Autodesk Fusion 360 part; units mm, degrees
(part 2 of 2)
  spline S384 degree 2 poles (40.9942, 8.1842) (40.8646, 8.1842) (40.7546, 8.116) knots 0 0 0 1 1 1
  spline S385 degree 2 poles (40.7546, 8.116) (40.6446, 8.0477) (40.5952, 7.9164) knots 0 0 0 1 1 1
  spline S386 degree 2 poles (40.5952, 7.9164) (40.5457, 7.7851) (40.5457, 7.5379) knots 0 0 0 1 1 1
  line L215 (40.5457, 7.5379) -> (40.5457, 6.5982)
  line L216 (40.5457, 6.5982) -> (40.2387, 6.5982)
  line L217 (44.3878, 7.1814) -> (44.705, 7.1422)
  spline S387 degree 2 poles (44.705, 7.1422) (44.6299, 6.8643) (44.427, 6.7108) knots 0 0 0 1 1 1
  spline S388 degree 2 poles (44.427, 6.7108) (44.2241, 6.5573) (43.9086, 6.5573) knots 0 0 0 1 1 1
  spline S389 degree 2 poles (43.9086, 6.5573) (43.5113, 6.5573) (43.2785, 6.802) knots 0 0 0 1 1 1
  spline S390 degree 2 poles (43.2785, 6.802) (43.0457, 7.0467) (43.0457, 7.4884) knots 0 0 0 1 1 1
  spline S391 degree 2 poles (43.0457, 7.4884) (43.0457, 7.9454) (43.281, 8.1978) knots 0 0 0 1 1 1
  spline S392 degree 2 poles (43.281, 8.1978) (43.5164, 8.4502) (43.8915, 8.4502) knots 0 0 0 1 1 1
  spline S393 degree 2 poles (43.8915, 8.4502) (44.2548, 8.4502) (44.485, 8.2029) knots 0 0 0 1 1 1
  spline S394 degree 2 poles (44.485, 8.2029) (44.7152, 7.9557) (44.7152, 7.5072) knots 0 0 0 1 1 1
  spline S395 degree 2 poles (44.7152, 7.5072) (44.7152, 7.4799) (44.7135, 7.4253) knots 0 0 0 1 1 1
  line L218 (44.7135, 7.4253) -> (43.3629, 7.4253)
  spline S396 degree 2 poles (43.3629, 7.4253) (43.3799, 7.1269) (43.5317, 6.9683) knots 0 0 0 1 1 1
  spline S397 degree 2 poles (43.5317, 6.9683) (43.6835, 6.8097) (43.9103, 6.8097) knots 0 0 0 1 1 1
  spline S398 degree 2 poles (43.9103, 6.8097) (44.0791, 6.8097) (44.1985, 6.8984) knots 0 0 0 1 1 1
  spline S399 degree 2 poles (44.1985, 6.8984) (44.3179, 6.987) (44.3878, 7.1814) knots 0 0 0 1 1 1
  line L219 (43.3799, 7.6777) -> (44.3912, 7.6777)
  spline S400 degree 2 poles (44.3912, 7.6777) (44.3707, 7.9062) (44.2752, 8.0205) knots 0 0 0 1 1 1
  spline S401 degree 2 poles (44.2752, 8.0205) (44.1286, 8.1978) (43.895, 8.1978) knots 0 0 0 1 1 1
  spline S402 degree 2 poles (43.895, 8.1978) (43.6835, 8.1978) (43.5394, 8.0563) knots 0 0 0 1 1 1
  spline S403 degree 2 poles (43.5394, 8.0563) (43.3953, 7.9147) (43.3799, 7.6777) knots 0 0 0 1 1 1
  line L220 (45.0904, 6.5982) -> (45.0904, 8.4093)
  line L221 (45.0904, 8.4093) -> (45.3666, 8.4093)
  line L222 (45.3666, 8.4093) -> (45.3666, 8.1518)
  spline S404 degree 2 poles (45.3666, 8.1518) (45.5662, 8.4502) (45.943, 8.4502) knots 0 0 0 1 1 1
  spline S405 degree 2 poles (45.943, 8.4502) (46.1068, 8.4502) (46.244, 8.3914) knots 0 0 0 1 1 1
  spline S406 degree 2 poles (46.244, 8.3914) (46.3813, 8.3325) (46.4495, 8.237) knots 0 0 0 1 1 1
  spline S407 degree 2 poles (46.4495, 8.237) (46.5177, 8.1415) (46.545, 8.0102) knots 0 0 0 1 1 1
  spline S408 degree 2 poles (46.545, 8.0102) (46.5621, 7.925) (46.5621, 7.7118) knots 0 0 0 1 1 1
  line L223 (46.5621, 7.7118) -> (46.5621, 6.5982)
  line L224 (46.5621, 6.5982) -> (46.2551, 6.5982)
  line L225 (46.2551, 6.5982) -> (46.2551, 7.6999)
  spline S409 degree 2 poles (46.2551, 7.6999) (46.2551, 7.8874) (46.2193, 7.9804) knots 0 0 0 1 1 1
  spline S410 degree 2 poles (46.2193, 7.9804) (46.1835, 8.0733) (46.0923, 8.1288) knots 0 0 0 1 1 1
  spline S411 degree 2 poles (46.0923, 8.1288) (46.001, 8.1842) (45.8782, 8.1842) knots 0 0 0 1 1 1
  spline S412 degree 2 poles (45.8782, 8.1842) (45.6821, 8.1842) (45.5397, 8.0597) knots 0 0 0 1 1 1
  spline S413 degree 2 poles (45.5397, 8.0597) (45.3973, 7.9352) (45.3973, 7.5873) knots 0 0 0 1 1 1
  line L226 (45.3973, 7.5873) -> (45.3973, 6.5982)
  line L227 (45.3973, 6.5982) -> (45.0904, 6.5982)
  line L228 (47.7029, 6.8728) -> (47.7473, 6.6016)
  spline S414 degree 2 poles (47.7473, 6.6016) (47.6177, 6.5744) (47.5153, 6.5744) knots 0 0 0 1 1 1
  spline S415 degree 2 poles (47.5153, 6.5744) (47.3482, 6.5744) (47.2561, 6.6272) knots 0 0 0 1 1 1
  spline S416 degree 2 poles (47.2561, 6.6272) (47.1641, 6.6801) (47.1265, 6.7662) knots 0 0 0 1 1 1
  spline S417 degree 2 poles (47.1265, 6.7662) (47.089, 6.8523) (47.089, 7.1286) knots 0 0 0 1 1 1
  line L229 (47.089, 7.1286) -> (47.089, 8.1705)
  line L230 (47.089, 8.1705) -> (46.8639, 8.1705)
  line L231 (46.8639, 8.1705) -> (46.8639, 8.4093)
  line L232 (46.8639, 8.4093) -> (47.089, 8.4093)
  line L233 (47.089, 8.4093) -> (47.089, 8.8578)
  line L234 (47.089, 8.8578) -> (47.3943, 9.042)
  line L235 (47.3943, 9.042) -> (47.3943, 8.4093)
  line L236 (47.3943, 8.4093) -> (47.7029, 8.4093)
  line L237 (47.7029, 8.4093) -> (47.7029, 8.1705)
  line L238 (47.7029, 8.1705) -> (47.3943, 8.1705)
  line L239 (47.3943, 8.1705) -> (47.3943, 7.1115)
  spline S418 degree 2 poles (47.3943, 7.1115) (47.3943, 6.9802) (47.4105, 6.9427) knots 0 0 0 1 1 1
  spline S419 degree 2 poles (47.4105, 6.9427) (47.4267, 6.9052) (47.4633, 6.883) knots 0 0 0 1 1 1
  spline S420 degree 2 poles (47.4633, 6.883) (47.5, 6.8608) (47.5682, 6.8608) knots 0 0 0 1 1 1
  spline S421 degree 2 poles (47.5682, 6.8608) (47.6194, 6.8608) (47.7029, 6.8728) knots 0 0 0 1 1 1
  line L240 (11.8426, 2.6965) -> (11.2884, 4.5075)
  line L241 (11.2884, 4.5075) -> (11.6056, 4.5075)
  line L242 (11.6056, 4.5075) -> (11.8938, 3.4621)
  line L243 (11.8938, 3.4621) -> (12.0012, 3.0733)
  spline S422 degree 2 poles (12.0012, 3.0733) (12.008, 3.1023) (12.095, 3.4468) knots 0 0 0 1 1 1
  line L244 (12.095, 3.4468) -> (12.3832, 4.5075)
  line L245 (12.3832, 4.5075) -> (12.6987, 4.5075)
  line L246 (12.6987, 4.5075) -> (12.9698, 3.457)
  line L247 (12.9698, 3.457) -> (13.0602, 3.1108)
  line L248 (13.0602, 3.1108) -> (13.1642, 3.4604)
  line L249 (13.1642, 3.4604) -> (13.4746, 4.5075)
  line L250 (13.4746, 4.5075) -> (13.773, 4.5075)
  line L251 (13.773, 4.5075) -> (13.2069, 2.6965)
  line L252 (13.2069, 2.6965) -> (12.888, 2.6965)
  line L253 (12.888, 2.6965) -> (12.5998, 3.781)
  line L254 (12.5998, 3.781) -> (12.5298, 4.0897)
  line L255 (12.5298, 4.0897) -> (12.1632, 2.6965)
  line L256 (12.1632, 2.6965) -> (11.8426, 2.6965)
  line L257 (14.3648, 2.6965) -> (13.8105, 4.5075)
  line L258 (13.8105, 4.5075) -> (14.1277, 4.5075)
  line L259 (14.1277, 4.5075) -> (14.4159, 3.4621)
  line L260 (14.4159, 3.4621) -> (14.5234, 3.0733)
  spline S423 degree 2 poles (14.5234, 3.0733) (14.5302, 3.1023) (14.6172, 3.4468) knots 0 0 0 1 1 1
  line L261 (14.6172, 3.4468) -> (14.9054, 4.5075)
  line L262 (14.9054, 4.5075) -> (15.2208, 4.5075)
  line L263 (15.2208, 4.5075) -> (15.492, 3.457)
  line L264 (15.492, 3.457) -> (15.5824, 3.1108)
  line L265 (15.5824, 3.1108) -> (15.6864, 3.4604)
  line L266 (15.6864, 3.4604) -> (15.9968, 4.5075)
  line L267 (15.9968, 4.5075) -> (16.2952, 4.5075)
  line L268 (16.2952, 4.5075) -> (15.729, 2.6965)
  line L269 (15.729, 2.6965) -> (15.4101, 2.6965)
  line L270 (15.4101, 2.6965) -> (15.1219, 3.781)
  line L271 (15.1219, 3.781) -> (15.052, 4.0897)
  line L272 (15.052, 4.0897) -> (14.6854, 2.6965)
  line L273 (14.6854, 2.6965) -> (14.3648, 2.6965)
  line L274 (16.8869, 2.6965) -> (16.3327, 4.5075)
  line L275 (16.3327, 4.5075) -> (16.6499, 4.5075)
  line L276 (16.6499, 4.5075) -> (16.9381, 3.4621)
  line L277 (16.9381, 3.4621) -> (17.0455, 3.0733)
  spline S424 degree 2 poles (17.0455, 3.0733) (17.0524, 3.1023) (17.1393, 3.4468) knots 0 0 0 1 1 1
  line L278 (17.1393, 3.4468) -> (17.4275, 4.5075)
  line L279 (17.4275, 4.5075) -> (17.743, 4.5075)
  line L280 (17.743, 4.5075) -> (18.0142, 3.457)
  line L281 (18.0142, 3.457) -> (18.1045, 3.1108)
  line L282 (18.1045, 3.1108) -> (18.2086, 3.4604)
  line L283 (18.2086, 3.4604) -> (18.5189, 4.5075)
  line L284 (18.5189, 4.5075) -> (18.8174, 4.5075)
  line L285 (18.8174, 4.5075) -> (18.2512, 2.6965)
  line L286 (18.2512, 2.6965) -> (17.9323, 2.6965)
  line L287 (17.9323, 2.6965) -> (17.6441, 3.781)
  line L288 (17.6441, 3.781) -> (17.5742, 4.0897)
  line L289 (17.5742, 4.0897) -> (17.2075, 2.6965)
  line L290 (17.2075, 2.6965) -> (16.8869, 2.6965)
  line L291 (18.9691, 2.6965) -> (18.9691, 3.046)
  line L292 (18.9691, 3.046) -> (19.3187, 3.046)
  line L293 (19.3187, 3.046) -> (19.3187, 2.6965)
  line L294 (19.3187, 2.6965) -> (18.9691, 2.6965)
  line L295 (19.8525, 2.6965) -> (19.8525, 4.5075)
  line L296 (19.8525, 4.5075) -> (20.127, 4.5075)
  line L297 (20.127, 4.5075) -> (20.127, 4.2534)
  spline S425 degree 2 poles (20.127, 4.2534) (20.2123, 4.3864) (20.3539, 4.4674) knots 0 0 0 1 1 1
  spline S426 degree 2 poles (20.3539, 4.4674) (20.4954, 4.5484) (20.6762, 4.5484) knots 0 0 0 1 1 1
  spline S427 degree 2 poles (20.6762, 4.5484) (20.8774, 4.5484) (21.0061, 4.4649) knots 0 0 0 1 1 1
  spline S428 degree 2 poles (21.0061, 4.4649) (21.1349, 4.3813) (21.1878, 4.2312) knots 0 0 0 1 1 1
  spline S429 degree 2 poles (21.1878, 4.2312) (21.4026, 4.5484) (21.7471, 4.5484) knots 0 0 0 1 1 1
  spline S430 degree 2 poles (21.7471, 4.5484) (22.0165, 4.5484) (22.1615, 4.3992) knots 0 0 0 1 1 1
  spline S431 degree 2 poles (22.1615, 4.3992) (22.3064, 4.25) (22.3064, 3.9396) knots 0 0 0 1 1 1
  line L298 (22.3064, 3.9396) -> (22.3064, 2.6965)
  line L299 (22.3064, 2.6965) -> (22.0012, 2.6965)
  line L300 (22.0012, 2.6965) -> (22.0012, 3.8373)
  spline S432 degree 2 poles (22.0012, 3.8373) (22.0012, 4.0215) (21.9713, 4.1025) knots 0 0 0 1 1 1
  spline S433 degree 2 poles (21.9713, 4.1025) (21.9415, 4.1835) (21.8631, 4.2329) knots 0 0 0 1 1 1
  spline S434 degree 2 poles (21.8631, 4.2329) (21.7846, 4.2824) (21.6789, 4.2824) knots 0 0 0 1 1 1
  spline S435 degree 2 poles (21.6789, 4.2824) (21.4879, 4.2824) (21.3617, 4.1554) knots 0 0 0 1 1 1
  spline S436 degree 2 poles (21.3617, 4.1554) (21.2355, 4.0283) (21.2355, 3.7486) knots 0 0 0 1 1 1
  line L301 (21.2355, 3.7486) -> (21.2355, 2.6965)
  line L302 (21.2355, 2.6965) -> (20.9285, 2.6965)
  line L303 (20.9285, 2.6965) -> (20.9285, 3.8731)
  spline S437 degree 2 poles (20.9285, 3.8731) (20.9285, 4.0778) (20.8535, 4.1801) knots 0 0 0 1 1 1
  spline S438 degree 2 poles (20.8535, 4.1801) (20.7785, 4.2824) (20.6079, 4.2824) knots 0 0 0 1 1 1
  spline S439 degree 2 poles (20.6079, 4.2824) (20.4783, 4.2824) (20.3683, 4.2142) knots 0 0 0 1 1 1
  spline S440 degree 2 poles (20.3683, 4.2142) (20.2584, 4.146) (20.2089, 4.0147) knots 0 0 0 1 1 1
  spline S441 degree 2 poles (20.2089, 4.0147) (20.1594, 3.8834) (20.1594, 3.6361) knots 0 0 0 1 1 1
  line L304 (20.1594, 3.6361) -> (20.1594, 2.6965)
  line L305 (20.1594, 2.6965) -> (19.8525, 2.6965)
  spline S442 degree 2 poles (22.6475, 3.602) (22.6475, 4.105) (22.9272, 4.3472) knots 0 0 0 1 1 1
  spline S443 degree 2 poles (22.9272, 4.3472) (23.1608, 4.5484) (23.4968, 4.5484) knots 0 0 0 1 1 1
  spline S444 degree 2 poles (23.4968, 4.5484) (23.8702, 4.5484) (24.1073, 4.3037) knots 0 0 0 1 1 1
  spline S445 degree 2 poles (24.1073, 4.3037) (24.3443, 4.059) (24.3443, 3.6276) knots 0 0 0 1 1 1
  spline S446 degree 2 poles (24.3443, 3.6276) (24.3443, 3.278) (24.2394, 3.0776) knots 0 0 0 1 1 1
  spline S447 degree 2 poles (24.2394, 3.0776) (24.1345, 2.8772) (23.9342, 2.7664) knots 0 0 0 1 1 1
  spline S448 degree 2 poles (23.9342, 2.7664) (23.7338, 2.6555) (23.4968, 2.6555) knots 0 0 0 1 1 1
  spline S449 degree 2 poles (23.4968, 2.6555) (23.1165, 2.6555) (22.882, 2.8994) knots 0 0 0 1 1 1
  spline S450 degree 2 poles (22.882, 2.8994) (22.6475, 3.1432) (22.6475, 3.602) knots 0 0 0 1 1 1
  spline S451 degree 2 poles (22.963, 3.602) (22.963, 3.2541) (23.1148, 3.081) knots 0 0 0 1 1 1
  spline S452 degree 2 poles (23.1148, 3.081) (23.2665, 2.9079) (23.4968, 2.9079) knots 0 0 0 1 1 1
  spline S453 degree 2 poles (23.4968, 2.9079) (23.7253, 2.9079) (23.877, 3.0819) knots 0 0 0 1 1 1
  spline S454 degree 2 poles (23.877, 3.0819) (24.0288, 3.2558) (24.0288, 3.6122) knots 0 0 0 1 1 1
  spline S455 degree 2 poles (24.0288, 3.6122) (24.0288, 3.9482) (23.8762, 4.1212) knots 0 0 0 1 1 1
  spline S456 degree 2 poles (23.8762, 4.1212) (23.7236, 4.2943) (23.4968, 4.2943) knots 0 0 0 1 1 1
  spline S457 degree 2 poles (23.4968, 4.2943) (23.2665, 4.2943) (23.1148, 4.1221) knots 0 0 0 1 1 1
  spline S458 degree 2 poles (23.1148, 4.1221) (22.963, 3.9499) (22.963, 3.602) knots 0 0 0 1 1 1
  line L306 (24.7041, 2.6965) -> (24.7041, 4.5075)
  line L307 (24.7041, 4.5075) -> (24.9804, 4.5075)
  line L308 (24.9804, 4.5075) -> (24.9804, 4.25)
  spline S459 degree 2 poles (24.9804, 4.25) (25.1799, 4.5484) (25.5568, 4.5484) knots 0 0 0 1 1 1
  spline S460 degree 2 poles (25.5568, 4.5484) (25.7205, 4.5484) (25.8578, 4.4896) knots 0 0 0 1 1 1
  spline S461 degree 2 poles (25.8578, 4.4896) (25.9951, 4.4308) (26.0633, 4.3353) knots 0 0 0 1 1 1
  spline S462 degree 2 poles (26.0633, 4.3353) (26.1315, 4.2398) (26.1588, 4.1085) knots 0 0 0 1 1 1
  spline S463 degree 2 poles (26.1588, 4.1085) (26.1758, 4.0232) (26.1758, 3.81) knots 0 0 0 1 1 1
  line L309 (26.1758, 3.81) -> (26.1758, 2.6965)
  line L310 (26.1758, 2.6965) -> (25.8689, 2.6965)
  line L311 (25.8689, 2.6965) -> (25.8689, 3.7981)
  spline S464 degree 2 poles (25.8689, 3.7981) (25.8689, 3.9857) (25.833, 4.0786) knots 0 0 0 1 1 1
  spline S465 degree 2 poles (25.833, 4.0786) (25.7972, 4.1716) (25.706, 4.227) knots 0 0 0 1 1 1
  spline S466 degree 2 poles (25.706, 4.227) (25.6148, 4.2824) (25.492, 4.2824) knots 0 0 0 1 1 1
  spline S467 degree 2 poles (25.492, 4.2824) (25.2959, 4.2824) (25.1535, 4.1579) knots 0 0 0 1 1 1
  spline S468 degree 2 poles (25.1535, 4.1579) (25.0111, 4.0334) (25.0111, 3.6855) knots 0 0 0 1 1 1
  line L312 (25.0111, 3.6855) -> (25.0111, 2.6965)
  line L313 (25.0111, 2.6965) -> (24.7041, 2.6965)
  line L314 (27.3167, 2.971) -> (27.361, 2.6999)
  spline S469 degree 2 poles (27.361, 2.6999) (27.2314, 2.6726) (27.1291, 2.6726) knots 0 0 0 1 1 1
  spline S470 degree 2 poles (27.1291, 2.6726) (26.962, 2.6726) (26.8699, 2.7254) knots 0 0 0 1 1 1
  spline S471 degree 2 poles (26.8699, 2.7254) (26.7778, 2.7783) (26.7403, 2.8644) knots 0 0 0 1 1 1
  spline S472 degree 2 poles (26.7403, 2.8644) (26.7028, 2.9505) (26.7028, 3.2268) knots 0 0 0 1 1 1
  line L315 (26.7028, 3.2268) -> (26.7028, 4.2688)
  line L316 (26.7028, 4.2688) -> (26.4777, 4.2688)
  line L317 (26.4777, 4.2688) -> (26.4777, 4.5075)
  line L318 (26.4777, 4.5075) -> (26.7028, 4.5075)
  line L319 (26.7028, 4.5075) -> (26.7028, 4.956)
  line L320 (26.7028, 4.956) -> (27.008, 5.1402)
  line L321 (27.008, 5.1402) -> (27.008, 4.5075)
  line L322 (27.008, 4.5075) -> (27.3167, 4.5075)
  line L323 (27.3167, 4.5075) -> (27.3167, 4.2688)
  line L324 (27.3167, 4.2688) -> (27.008, 4.2688)
  line L325 (27.008, 4.2688) -> (27.008, 3.2098)
  spline S473 degree 2 poles (27.008, 3.2098) (27.008, 3.0784) (27.0242, 3.0409) knots 0 0 0 1 1 1
  spline S474 degree 2 poles (27.0242, 3.0409) (27.0404, 3.0034) (27.0771, 2.9812) knots 0 0 0 1 1 1
  spline S475 degree 2 poles (27.0771, 2.9812) (27.1137, 2.9591) (27.182, 2.9591) knots 0 0 0 1 1 1
  spline S476 degree 2 poles (27.182, 2.9591) (27.2331, 2.9591) (27.3167, 2.971) knots 0 0 0 1 1 1
  line L326 (28.8566, 3.2797) -> (29.1738, 3.2405)
  spline S477 degree 2 poles (29.1738, 3.2405) (29.0987, 2.9625) (28.8958, 2.809) knots 0 0 0 1 1 1
  spline S478 degree 2 poles (28.8958, 2.809) (28.6929, 2.6555) (28.3774, 2.6555) knots 0 0 0 1 1 1
  spline S479 degree 2 poles (28.3774, 2.6555) (27.98, 2.6555) (27.7473, 2.9002) knots 0 0 0 1 1 1
  spline S480 degree 2 poles (27.7473, 2.9002) (27.5145, 3.145) (27.5145, 3.5866) knots 0 0 0 1 1 1
  spline S481 degree 2 poles (27.5145, 3.5866) (27.5145, 4.0437) (27.7498, 4.296) knots 0 0 0 1 1 1
  spline S482 degree 2 poles (27.7498, 4.296) (27.9852, 4.5484) (28.3603, 4.5484) knots 0 0 0 1 1 1
  spline S483 degree 2 poles (28.3603, 4.5484) (28.7236, 4.5484) (28.9538, 4.3012) knots 0 0 0 1 1 1
  spline S484 degree 2 poles (28.9538, 4.3012) (29.184, 4.0539) (29.184, 3.6054) knots 0 0 0 1 1 1
  spline S485 degree 2 poles (29.184, 3.6054) (29.184, 3.5781) (29.1823, 3.5235) knots 0 0 0 1 1 1
  line L327 (29.1823, 3.5235) -> (27.8317, 3.5235)
  spline S486 degree 2 poles (27.8317, 3.5235) (27.8487, 3.2251) (28.0005, 3.0665) knots 0 0 0 1 1 1
  spline S487 degree 2 poles (28.0005, 3.0665) (28.1523, 2.9079) (28.3791, 2.9079) knots 0 0 0 1 1 1
  spline S488 degree 2 poles (28.3791, 2.9079) (28.5479, 2.9079) (28.6673, 2.9966) knots 0 0 0 1 1 1
  spline S489 degree 2 poles (28.6673, 2.9966) (28.7867, 3.0853) (28.8566, 3.2797) knots 0 0 0 1 1 1
  line L328 (27.8487, 3.7759) -> (28.86, 3.7759)
  spline S490 degree 2 poles (28.86, 3.7759) (28.8395, 4.0044) (28.744, 4.1187) knots 0 0 0 1 1 1
  spline S491 degree 2 poles (28.744, 4.1187) (28.5974, 4.296) (28.3637, 4.296) knots 0 0 0 1 1 1
  spline S492 degree 2 poles (28.3637, 4.296) (28.1523, 4.296) (28.0082, 4.1545) knots 0 0 0 1 1 1
  spline S493 degree 2 poles (28.0082, 4.1545) (27.8641, 4.013) (27.8487, 3.7759) knots 0 0 0 1 1 1
  line L329 (30.7341, 2.6965) -> (30.7341, 2.925)
  spline S494 degree 2 poles (30.7341, 2.925) (30.5619, 2.6555) (30.2277, 2.6555) knots 0 0 0 1 1 1
  spline S495 degree 2 poles (30.2277, 2.6555) (30.0111, 2.6555) (29.8295, 2.7749) knots 0 0 0 1 1 1
  spline S496 degree 2 poles (29.8295, 2.7749) (29.6479, 2.8943) (29.5481, 3.1083) knots 0 0 0 1 1 1
  spline S497 degree 2 poles (29.5481, 3.1083) (29.4483, 3.3223) (29.4483, 3.6003) knots 0 0 0 1 1 1
  spline S498 degree 2 poles (29.4483, 3.6003) (29.4483, 3.8714) (29.5387, 4.0923) knots 0 0 0 1 1 1
  spline S499 degree 2 poles (29.5387, 4.0923) (29.6291, 4.3131) (29.8099, 4.4308) knots 0 0 0 1 1 1
  spline S500 degree 2 poles (29.8099, 4.4308) (29.9906, 4.5484) (30.214, 4.5484) knots 0 0 0 1 1 1
  spline S501 degree 2 poles (30.214, 4.5484) (30.3777, 4.5484) (30.5056, 4.4794) knots 0 0 0 1 1 1
  spline S502 degree 2 poles (30.5056, 4.4794) (30.6335, 4.4103) (30.7137, 4.2995) knots 0 0 0 1 1 1
  line L330 (30.7137, 4.2995) -> (30.7137, 5.1965)
  line L331 (30.7137, 5.1965) -> (31.0189, 5.1965)
  line L332 (31.0189, 5.1965) -> (31.0189, 2.6965)
  line L333 (31.0189, 2.6965) -> (30.7341, 2.6965)
  spline S503 degree 2 poles (29.7638, 3.6003) (29.7638, 3.2524) (29.9105, 3.0801) knots 0 0 0 1 1 1
  spline S504 degree 2 poles (29.9105, 3.0801) (30.0571, 2.9079) (30.2566, 2.9079) knots 0 0 0 1 1 1
  spline S505 degree 2 poles (30.2566, 2.9079) (30.4579, 2.9079) (30.5986, 3.0725) knots 0 0 0 1 1 1
  spline S506 degree 2 poles (30.5986, 3.0725) (30.7393, 3.237) (30.7393, 3.5747) knots 0 0 0 1 1 1
  spline S507 degree 2 poles (30.7393, 3.5747) (30.7393, 3.9465) (30.596, 4.1204) knots 0 0 0 1 1 1
  spline S508 degree 2 poles (30.596, 4.1204) (30.4528, 4.2943) (30.243, 4.2943) knots 0 0 0 1 1 1
  spline S509 degree 2 poles (30.243, 4.2943) (30.0384, 4.2943) (29.9011, 4.1272) knots 0 0 0 1 1 1
  spline S510 degree 2 poles (29.9011, 4.1272) (29.7638, 3.9601) (29.7638, 3.6003) knots 0 0 0 1 1 1
  line L334 (32.7413, 3.2797) -> (33.0585, 3.2405)
  spline S511 degree 2 poles (33.0585, 3.2405) (32.9835, 2.9625) (32.7805, 2.809) knots 0 0 0 1 1 1
  spline S512 degree 2 poles (32.7805, 2.809) (32.5776, 2.6555) (32.2621, 2.6555) knots 0 0 0 1 1 1
  spline S513 degree 2 poles (32.2621, 2.6555) (31.8648, 2.6555) (31.632, 2.9002) knots 0 0 0 1 1 1
  spline S514 degree 2 poles (31.632, 2.9002) (31.3992, 3.145) (31.3992, 3.5866) knots 0 0 0 1 1 1
  spline S515 degree 2 poles (31.3992, 3.5866) (31.3992, 4.0437) (31.6345, 4.296) knots 0 0 0 1 1 1
  spline S516 degree 2 poles (31.6345, 4.296) (31.8699, 4.5484) (32.2451, 4.5484) knots 0 0 0 1 1 1
  spline S517 degree 2 poles (32.2451, 4.5484) (32.6083, 4.5484) (32.8385, 4.3012) knots 0 0 0 1 1 1
  spline S518 degree 2 poles (32.8385, 4.3012) (33.0687, 4.0539) (33.0687, 3.6054) knots 0 0 0 1 1 1
  spline S519 degree 2 poles (33.0687, 3.6054) (33.0687, 3.5781) (33.067, 3.5235) knots 0 0 0 1 1 1
  line L335 (33.067, 3.5235) -> (31.7164, 3.5235)
  spline S520 degree 2 poles (31.7164, 3.5235) (31.7335, 3.2251) (31.8852, 3.0665) knots 0 0 0 1 1 1
  spline S521 degree 2 poles (31.8852, 3.0665) (32.037, 2.9079) (32.2638, 2.9079) knots 0 0 0 1 1 1
  spline S522 degree 2 poles (32.2638, 2.9079) (32.4326, 2.9079) (32.552, 2.9966) knots 0 0 0 1 1 1
  spline S523 degree 2 poles (32.552, 2.9966) (32.6714, 3.0853) (32.7413, 3.2797) knots 0 0 0 1 1 1
  line L336 (31.7335, 3.7759) -> (32.7447, 3.7759)
  spline S524 degree 2 poles (32.7447, 3.7759) (32.7243, 4.0044) (32.6288, 4.1187) knots 0 0 0 1 1 1
  spline S525 degree 2 poles (32.6288, 4.1187) (32.4821, 4.296) (32.2485, 4.296) knots 0 0 0 1 1 1
  spline S526 degree 2 poles (32.2485, 4.296) (32.037, 4.296) (31.8929, 4.1545) knots 0 0 0 1 1 1
  spline S527 degree 2 poles (31.8929, 4.1545) (31.7488, 4.013) (31.7335, 3.7759) knots 0 0 0 1 1 1
  line L337 (33.4371, 2.6965) -> (33.4371, 5.1965)
  line L338 (33.4371, 5.1965) -> (33.744, 5.1965)
  line L339 (33.744, 5.1965) -> (33.744, 2.6965)
  line L340 (33.744, 2.6965) -> (33.4371, 2.6965)
  line L341 (34.1635, 2.5464) -> (34.462, 2.502)
  spline S528 degree 2 poles (34.462, 2.502) (34.4807, 2.3639) (34.566, 2.3008) knots 0 0 0 1 1 1
  spline S529 degree 2 poles (34.566, 2.3008) (34.6803, 2.2156) (34.8781, 2.2156) knots 0 0 0 1 1 1
  spline S530 degree 2 poles (34.8781, 2.2156) (35.0912, 2.2156) (35.2072, 2.3008) knots 0 0 0 1 1 1
  spline S531 degree 2 poles (35.2072, 2.3008) (35.3232, 2.3861) (35.3641, 2.5396) knots 0 0 0 1 1 1
  spline S532 degree 2 poles (35.3641, 2.5396) (35.388, 2.6334) (35.3863, 2.9335) knots 0 0 0 1 1 1
  spline S533 degree 2 poles (35.3863, 2.9335) (35.185, 2.6965) (34.8849, 2.6965) knots 0 0 0 1 1 1
  spline S534 degree 2 poles (34.8849, 2.6965) (34.5114, 2.6965) (34.3068, 2.9659) knots 0 0 0 1 1 1
  spline S535 degree 2 poles (34.3068, 2.9659) (34.1021, 3.2353) (34.1021, 3.6122) knots 0 0 0 1 1 1
  spline S536 degree 2 poles (34.1021, 3.6122) (34.1021, 3.8714) (34.1959, 4.0906) knots 0 0 0 1 1 1
  spline S537 degree 2 poles (34.1959, 4.0906) (34.2897, 4.3097) (34.4679, 4.4291) knots 0 0 0 1 1 1
  spline S538 degree 2 poles (34.4679, 4.4291) (34.6461, 4.5484) (34.8866, 4.5484) knots 0 0 0 1 1 1
  spline S539 degree 2 poles (34.8866, 4.5484) (35.2072, 4.5484) (35.4152, 4.2892) knots 0 0 0 1 1 1
  line L342 (35.4152, 4.2892) -> (35.4152, 4.5075)
  line L343 (35.4152, 4.5075) -> (35.6983, 4.5075)
  line L344 (35.6983, 4.5075) -> (35.6983, 2.942)
  spline S540 degree 2 poles (35.6983, 2.942) (35.6983, 2.5191) (35.6122, 2.3426) knots 0 0 0 1 1 1
  spline S541 degree 2 poles (35.6122, 2.3426) (35.5261, 2.1661) (35.3394, 2.0638) knots 0 0 0 1 1 1
  spline S542 degree 2 poles (35.3394, 2.0638) (35.1526, 1.9615) (34.8798, 1.9615) knots 0 0 0 1 1 1
  spline S543 degree 2 poles (34.8798, 1.9615) (34.5558, 1.9615) (34.3562, 2.1073) knots 0 0 0 1 1 1
  spline S544 degree 2 poles (34.3562, 2.1073) (34.1567, 2.2531) (34.1635, 2.5464) knots 0 0 0 1 1 1
  spline S545 degree 2 poles (34.4176, 3.6344) (34.4176, 3.278) (34.5592, 3.1143) knots 0 0 0 1 1 1
  spline S546 degree 2 poles (34.5592, 3.1143) (34.7007, 2.9505) (34.9139, 2.9505) knots 0 0 0 1 1 1
  spline S547 degree 2 poles (34.9139, 2.9505) (35.1253, 2.9505) (35.2686, 3.1134) knots 0 0 0 1 1 1
  spline S548 degree 2 poles (35.2686, 3.1134) (35.4118, 3.2763) (35.4118, 3.6241) knots 0 0 0 1 1 1
  spline S549 degree 2 poles (35.4118, 3.6241) (35.4118, 3.9567) (35.2643, 4.1255) knots 0 0 0 1 1 1
  spline S550 degree 2 poles (35.2643, 4.1255) (35.1168, 4.2943) (34.9088, 4.2943) knots 0 0 0 1 1 1
  spline S551 degree 2 poles (34.9088, 4.2943) (34.7041, 4.2943) (34.5609, 4.1281) knots 0 0 0 1 1 1
  spline S552 degree 2 poles (34.5609, 4.1281) (34.4176, 3.9618) (34.4176, 3.6344) knots 0 0 0 1 1 1
  spline S553 degree 2 poles (37.344, 2.9199) (37.1734, 2.7749) (37.0157, 2.7152) knots 0 0 0 1 1 1
  spline S554 degree 2 poles (37.0157, 2.7152) (36.8579, 2.6555) (36.6772, 2.6555) knots 0 0 0 1 1 1
  spline S555 degree 2 poles (36.6772, 2.6555) (36.3787, 2.6555) (36.2185, 2.8013) knots 0 0 0 1 1 1
  spline S556 degree 2 poles (36.2185, 2.8013) (36.0582, 2.9471) (36.0582, 3.1739) knots 0 0 0 1 1 1
  spline S557 degree 2 poles (36.0582, 3.1739) (36.0582, 3.307) (36.1187, 3.417) knots 0 0 0 1 1 1
  spline S558 degree 2 poles (36.1187, 3.417) (36.1792, 3.5269) (36.2773, 3.5935) knots 0 0 0 1 1 1
  spline S559 degree 2 poles (36.2773, 3.5935) (36.3753, 3.66) (36.4981, 3.6941) knots 0 0 0 1 1 1
  spline S560 degree 2 poles (36.4981, 3.6941) (36.5885, 3.7179) (36.771, 3.7401) knots 0 0 0 1 1 1
  spline S561 degree 2 poles (36.771, 3.7401) (37.1427, 3.7844) (37.3184, 3.8458) knots 0 0 0 1 1 1
  spline S562 degree 2 poles (37.3184, 3.8458) (37.3201, 3.9089) (37.3201, 3.926) knots 0 0 0 1 1 1
  spline S563 degree 2 poles (37.3201, 3.926) (37.3201, 4.1136) (37.2331, 4.1903) knots 0 0 0 1 1 1
  spline S564 degree 2 poles (37.2331, 4.1903) (37.1154, 4.2943) (36.8835, 4.2943) knots 0 0 0 1 1 1
  spline S565 degree 2 poles (36.8835, 4.2943) (36.6669, 4.2943) (36.5638, 4.2185) knots 0 0 0 1 1 1
  spline S566 degree 2 poles (36.5638, 4.2185) (36.4606, 4.1426) (36.4112, 3.9499) knots 0 0 0 1 1 1
  line L345 (36.4112, 3.9499) -> (36.111, 3.9908)
  spline S567 degree 2 poles (36.111, 3.9908) (36.1519, 4.1835) (36.2457, 4.302) knots 0 0 0 1 1 1
  spline S568 degree 2 poles (36.2457, 4.302) (36.3395, 4.4205) (36.5169, 4.4845) knots 0 0 0 1 1 1
  spline S569 degree 2 poles (36.5169, 4.4845) (36.6942, 4.5484) (36.9279, 4.5484) knots 0 0 0 1 1 1
  spline S570 degree 2 poles (36.9279, 4.5484) (37.1598, 4.5484) (37.3047, 4.4939) knots 0 0 0 1 1 1
  spline S571 degree 2 poles (37.3047, 4.4939) (37.4497, 4.4393) (37.5179, 4.3566) knots 0 0 0 1 1 1
  spline S572 degree 2 poles (37.5179, 4.3566) (37.5861, 4.2739) (37.6134, 4.1477) knots 0 0 0 1 1 1
  spline S573 degree 2 poles (37.6134, 4.1477) (37.6287, 4.0692) (37.6287, 3.8646) knots 0 0 0 1 1 1
  line L346 (37.6287, 3.8646) -> (37.6287, 3.4553)
  spline S574 degree 2 poles (37.6287, 3.4553) (37.6287, 3.0273) (37.6484, 2.9139) knots 0 0 0 1 1 1
  spline S575 degree 2 poles (37.6484, 2.9139) (37.668, 2.8005) (37.726, 2.6965) knots 0 0 0 1 1 1
  line L347 (37.726, 2.6965) -> (37.4054, 2.6965)
  spline S576 degree 2 poles (37.4054, 2.6965) (37.3576, 2.792) (37.344, 2.9199) knots 0 0 0 1 1 1
  spline S577 degree 2 poles (37.3184, 3.6054) (37.1513, 3.5372) (36.817, 3.4894) knots 0 0 0 1 1 1
  spline S578 degree 2 poles (36.817, 3.4894) (36.6277, 3.4621) (36.5493, 3.428) knots 0 0 0 1 1 1
  spline S579 degree 2 poles (36.5493, 3.428) (36.4708, 3.3939) (36.4282, 3.3283) knots 0 0 0 1 1 1
  spline S580 degree 2 poles (36.4282, 3.3283) (36.3856, 3.2626) (36.3856, 3.1825) knots 0 0 0 1 1 1
  spline S581 degree 2 poles (36.3856, 3.1825) (36.3856, 3.0597) (36.4785, 2.9778) knots 0 0 0 1 1 1
  spline S582 degree 2 poles (36.4785, 2.9778) (36.5715, 2.896) (36.7505, 2.896) knots 0 0 0 1 1 1
  spline S583 degree 2 poles (36.7505, 2.896) (36.9279, 2.896) (37.066, 2.9736) knots 0 0 0 1 1 1
  spline S584 degree 2 poles (37.066, 2.9736) (37.2041, 3.0512) (37.2689, 3.1859) knots 0 0 0 1 1 1
  spline S585 degree 2 poles (37.2689, 3.1859) (37.3184, 3.2899) (37.3184, 3.4928) knots 0 0 0 1 1 1
  line L348 (37.3184, 3.4928) -> (37.3184, 3.6054)
  line L349 (38.0977, 2.6965) -> (38.0977, 5.1965)
  line L350 (38.0977, 5.1965) -> (38.4047, 5.1965)
  line L351 (38.4047, 5.1965) -> (38.4047, 2.6965)
  line L352 (38.4047, 2.6965) -> (38.0977, 2.6965)
  line L353 (38.8736, 2.6965) -> (38.8736, 5.1965)
  line L354 (38.8736, 5.1965) -> (39.1806, 5.1965)
  line L355 (39.1806, 5.1965) -> (39.1806, 2.6965)
  line L356 (39.1806, 2.6965) -> (38.8736, 2.6965)
  spline S586 degree 2 poles (39.5421, 3.602) (39.5421, 4.105) (39.8218, 4.3472) knots 0 0 0 1 1 1
  spline S587 degree 2 poles (39.8218, 4.3472) (40.0554, 4.5484) (40.3914, 4.5484) knots 0 0 0 1 1 1
  spline S588 degree 2 poles (40.3914, 4.5484) (40.7648, 4.5484) (41.0019, 4.3037) knots 0 0 0 1 1 1
  spline S589 degree 2 poles (41.0019, 4.3037) (41.2389, 4.059) (41.2389, 3.6276) knots 0 0 0 1 1 1
  spline S590 degree 2 poles (41.2389, 3.6276) (41.2389, 3.278) (41.134, 3.0776) knots 0 0 0 1 1 1
  spline S591 degree 2 poles (41.134, 3.0776) (41.0292, 2.8772) (40.8288, 2.7664) knots 0 0 0 1 1 1
  spline S592 degree 2 poles (40.8288, 2.7664) (40.6284, 2.6555) (40.3914, 2.6555) knots 0 0 0 1 1 1
  spline S593 degree 2 poles (40.3914, 2.6555) (40.0111, 2.6555) (39.7766, 2.8994) knots 0 0 0 1 1 1
  spline S594 degree 2 poles (39.7766, 2.8994) (39.5421, 3.1432) (39.5421, 3.602) knots 0 0 0 1 1 1
  spline S595 degree 2 poles (39.8576, 3.602) (39.8576, 3.2541) (40.0094, 3.081) knots 0 0 0 1 1 1
  spline S596 degree 2 poles (40.0094, 3.081) (40.1612, 2.9079) (40.3914, 2.9079) knots 0 0 0 1 1 1
  spline S597 degree 2 poles (40.3914, 2.9079) (40.6199, 2.9079) (40.7717, 3.0819) knots 0 0 0 1 1 1
  spline S598 degree 2 poles (40.7717, 3.0819) (40.9234, 3.2558) (40.9234, 3.6122) knots 0 0 0 1 1 1
  spline S599 degree 2 poles (40.9234, 3.6122) (40.9234, 3.9482) (40.7708, 4.1212) knots 0 0 0 1 1 1
  spline S600 degree 2 poles (40.7708, 4.1212) (40.6182, 4.2943) (40.3914, 4.2943) knots 0 0 0 1 1 1
  spline S601 degree 2 poles (40.3914, 4.2943) (40.1612, 4.2943) (40.0094, 4.1221) knots 0 0 0 1 1 1
  spline S602 degree 2 poles (40.0094, 4.1221) (39.8576, 3.9499) (39.8576, 3.602) knots 0 0 0 1 1 1
  line L357 (41.6857, 2.6965) -> (41.6857, 3.046)
  line L358 (41.6857, 3.046) -> (42.0353, 3.046)
  line L359 (42.0353, 3.046) -> (42.0353, 2.6965)
  line L360 (42.0353, 2.6965) -> (41.6857, 2.6965)
  line L361 (43.7509, 3.3598) -> (44.0527, 3.3206)
  spline S603 degree 2 poles (44.0527, 3.3206) (44.0032, 3.0085) (43.7995, 2.832) knots 0 0 0 1 1 1
  spline S604 degree 2 poles (43.7995, 2.832) (43.5957, 2.6555) (43.2989, 2.6555) knots 0 0 0 1 1 1
  spline S605 degree 2 poles (43.2989, 2.6555) (42.9272, 2.6555) (42.7012, 2.8985) knots 0 0 0 1 1 1
  spline S606 degree 2 poles (42.7012, 2.8985) (42.4753, 3.1415) (42.4753, 3.5952) knots 0 0 0 1 1 1
  spline S607 degree 2 poles (42.4753, 3.5952) (42.4753, 3.8885) (42.5725, 4.1085) knots 0 0 0 1 1 1
  spline S608 degree 2 poles (42.5725, 4.1085) (42.6697, 4.3284) (42.8683, 4.4384) knots 0 0 0 1 1 1
  spline S609 degree 2 poles (42.8683, 4.4384) (43.067, 4.5484) (43.3006, 4.5484) knots 0 0 0 1 1 1
  spline S610 degree 2 poles (43.3006, 4.5484) (43.5957, 4.5484) (43.7833, 4.3992) knots 0 0 0 1 1 1
  spline S611 degree 2 poles (43.7833, 4.3992) (43.9708, 4.25) (44.0237, 3.9754) knots 0 0 0 1 1 1
  line L362 (44.0237, 3.9754) -> (43.7253, 3.9294)
  spline S612 degree 2 poles (43.7253, 3.9294) (43.6826, 4.1119) (43.5744, 4.204) knots 0 0 0 1 1 1
  spline S613 degree 2 poles (43.5744, 4.204) (43.4661, 4.296) (43.3126, 4.296) knots 0 0 0 1 1 1
  spline S614 degree 2 poles (43.3126, 4.296) (43.0807, 4.296) (42.9357, 4.1298) knots 0 0 0 1 1 1
  spline S615 degree 2 poles (42.9357, 4.1298) (42.7908, 3.9635) (42.7908, 3.6037) knots 0 0 0 1 1 1
  spline S616 degree 2 poles (42.7908, 3.6037) (42.7908, 3.2387) (42.9306, 3.0733) knots 0 0 0 1 1 1
  spline S617 degree 2 poles (42.9306, 3.0733) (43.0704, 2.9079) (43.2955, 2.9079) knots 0 0 0 1 1 1
  spline S618 degree 2 poles (43.2955, 2.9079) (43.4763, 2.9079) (43.5974, 3.0188) knots 0 0 0 1 1 1
  spline S619 degree 2 poles (43.5974, 3.0188) (43.7185, 3.1296) (43.7509, 3.3598) knots 0 0 0 1 1 1
  spline S620 degree 2 poles (44.2011, 3.602) (44.2011, 4.105) (44.4807, 4.3472) knots 0 0 0 1 1 1
  spline S621 degree 2 poles (44.4807, 4.3472) (44.7144, 4.5484) (45.0503, 4.5484) knots 0 0 0 1 1 1
  spline S622 degree 2 poles (45.0503, 4.5484) (45.4238, 4.5484) (45.6608, 4.3037) knots 0 0 0 1 1 1
  spline S623 degree 2 poles (45.6608, 4.3037) (45.8978, 4.059) (45.8978, 3.6276) knots 0 0 0 1 1 1
  spline S624 degree 2 poles (45.8978, 3.6276) (45.8978, 3.278) (45.793, 3.0776) knots 0 0 0 1 1 1
  spline S625 degree 2 poles (45.793, 3.0776) (45.6881, 2.8772) (45.4877, 2.7664) knots 0 0 0 1 1 1
  spline S626 degree 2 poles (45.4877, 2.7664) (45.2873, 2.6555) (45.0503, 2.6555) knots 0 0 0 1 1 1
  spline S627 degree 2 poles (45.0503, 2.6555) (44.67, 2.6555) (44.4355, 2.8994) knots 0 0 0 1 1 1
  spline S628 degree 2 poles (44.4355, 2.8994) (44.2011, 3.1432) (44.2011, 3.602) knots 0 0 0 1 1 1
  spline S629 degree 2 poles (44.5165, 3.602) (44.5165, 3.2541) (44.6683, 3.081) knots 0 0 0 1 1 1
  spline S630 degree 2 poles (44.6683, 3.081) (44.8201, 2.9079) (45.0503, 2.9079) knots 0 0 0 1 1 1
  spline S631 degree 2 poles (45.0503, 2.9079) (45.2788, 2.9079) (45.4306, 3.0819) knots 0 0 0 1 1 1
  spline S632 degree 2 poles (45.4306, 3.0819) (45.5824, 3.2558) (45.5824, 3.6122) knots 0 0 0 1 1 1
  spline S633 degree 2 poles (45.5824, 3.6122) (45.5824, 3.9482) (45.4297, 4.1212) knots 0 0 0 1 1 1
  spline S634 degree 2 poles (45.4297, 4.1212) (45.2771, 4.2943) (45.0503, 4.2943) knots 0 0 0 1 1 1
  spline S635 degree 2 poles (45.0503, 4.2943) (44.8201, 4.2943) (44.6683, 4.1221) knots 0 0 0 1 1 1
  spline S636 degree 2 poles (44.6683, 4.1221) (44.5165, 3.9499) (44.5165, 3.602) knots 0 0 0 1 1 1
  line L363 (46.2577, 2.6965) -> (46.2577, 4.5075)
  line L364 (46.2577, 4.5075) -> (46.5322, 4.5075)
  line L365 (46.5322, 4.5075) -> (46.5322, 4.2534)
  spline S637 degree 2 poles (46.5322, 4.2534) (46.6175, 4.3864) (46.759, 4.4674) knots 0 0 0 1 1 1
  spline S638 degree 2 poles (46.759, 4.4674) (46.9006, 4.5484) (47.0813, 4.5484) knots 0 0 0 1 1 1
  spline S639 degree 2 poles (47.0813, 4.5484) (47.2826, 4.5484) (47.4113, 4.4649) knots 0 0 0 1 1 1
  spline S640 degree 2 poles (47.4113, 4.4649) (47.5401, 4.3813) (47.5929, 4.2312) knots 0 0 0 1 1 1
  spline S641 degree 2 poles (47.5929, 4.2312) (47.8078, 4.5484) (48.1523, 4.5484) knots 0 0 0 1 1 1
  spline S642 degree 2 poles (48.1523, 4.5484) (48.4217, 4.5484) (48.5667, 4.3992) knots 0 0 0 1 1 1
  spline S643 degree 2 poles (48.5667, 4.3992) (48.7116, 4.25) (48.7116, 3.9396) knots 0 0 0 1 1 1
  line L366 (48.7116, 3.9396) -> (48.7116, 2.6965)
  line L367 (48.7116, 2.6965) -> (48.4064, 2.6965)
  line L368 (48.4064, 2.6965) -> (48.4064, 3.8373)
  spline S644 degree 2 poles (48.4064, 3.8373) (48.4064, 4.0215) (48.3765, 4.1025) knots 0 0 0 1 1 1
  spline S645 degree 2 poles (48.3765, 4.1025) (48.3467, 4.1835) (48.2682, 4.2329) knots 0 0 0 1 1 1
  spline S646 degree 2 poles (48.2682, 4.2329) (48.1898, 4.2824) (48.0841, 4.2824) knots 0 0 0 1 1 1
  spline S647 degree 2 poles (48.0841, 4.2824) (47.8931, 4.2824) (47.7669, 4.1554) knots 0 0 0 1 1 1
  spline S648 degree 2 poles (47.7669, 4.1554) (47.6407, 4.0283) (47.6407, 3.7486) knots 0 0 0 1 1 1
  line L369 (47.6407, 3.7486) -> (47.6407, 2.6965)
  line L370 (47.6407, 2.6965) -> (47.3337, 2.6965)
  line L371 (47.3337, 2.6965) -> (47.3337, 3.8731)
  spline S649 degree 2 poles (47.3337, 3.8731) (47.3337, 4.0778) (47.2587, 4.1801) knots 0 0 0 1 1 1
  spline S650 degree 2 poles (47.2587, 4.1801) (47.1837, 4.2824) (47.0131, 4.2824) knots 0 0 0 1 1 1
  spline S651 degree 2 poles (47.0131, 4.2824) (46.8835, 4.2824) (46.7735, 4.2142) knots 0 0 0 1 1 1
  spline S652 degree 2 poles (46.7735, 4.2142) (46.6635, 4.146) (46.6141, 4.0147) knots 0 0 0 1 1 1
  spline S653 degree 2 poles (46.6141, 4.0147) (46.5646, 3.8834) (46.5646, 3.6361) knots 0 0 0 1 1 1
  line L372 (46.5646, 3.6361) -> (46.5646, 2.6965)
  line L373 (46.5646, 2.6965) -> (46.2577, 2.6965)
  circle A0 centre (4, 31) radius 2.5
  dimension "d2" = 60
  dimension "d3" = 1
  dimension "d5" = 35
  dimension "d7" = 5
  constraint parallel L0 L2
  constraint coincident L0 L3.end
  constraint perpendicular L1 L3
  constraint perpendicular L6 L7
  constraint parallel L5 L8
  constraint perpendicular L8 L9
  constraint coincident L9 L10.start
  constraint perpendicular L9 L10
  constraint coincident L9 L11.end
  constraint coincident L7 L11.end
  constraint coincident L6 L12.end
  constraint coincident L12 L13.start
  constraint vertical L13
  constraint coincident L6 L14.end
  constraint parallel L12 L14
  constraint coincident L5 L15.start
  constraint perpendicular L5 L15
  constraint perpendicular L15 L16
  constraint perpendicular L16 L17
  constraint horizontal L18
  constraint perpendicular L16 L19
  constraint parallel L18 L20
  constraint coincident L5 L21.end
  constraint perpendicular L5 L21
  constraint parallel L19 L22
  constraint coincident L5 L23.end
  constraint vertical L23
  constraint perpendicular L5 L24
  constraint perpendicular L5 L25
  constraint coincident L21 L27.end
  constraint parallel L20 L27
  constraint coincident L21 L28.start
  constraint horizontal L28
  constraint horizontal L30
  constraint parallel L30 L32
  constraint parallel L32 L34
  constraint coincident L5 L36.end
  constraint parallel L34 L36
  constraint coincident L37 L39.end
  constraint coincident L5 L42.start
  constraint coincident L9.end L12
  constraint horizontal L43
  constraint coincident L0.start L43
  constraint perpendicular L16 L45
  constraint coincident L5 L46.end
  constraint vertical L46
  constraint coincident L44 L47.start
  constraint horizontal L48
  constraint vertical L49
  constraint horizontal L50
  constraint vertical L51
  constraint perpendicular L43 L54
  measures "d2" distance of L48.start L48.end
  measures "d5" distance of L48 L50
  measures "d7" diameter of A0
extrude "Estrusione1" add sketch "Schizzo1" along normal blind 2 contours L48 L49 L50 L51
